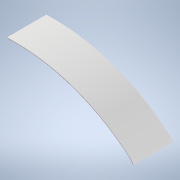
# Autodesk Inventor part: Hood Lexan
Saved by Autodesk Inventor 2022 (Build 260153070, 153G)
## iProperties
Created: 2021-09-03
Part Number: Hood Lexan
Material: Polycarbonate, Clear
Document SubType Name: Modeling
Designer: Main Account
Density: 1.2 g/cm^3
Appearance: Polycarbonate - Clear
Author: Main Account
Autodesk Inventor part; units mm, degrees
ref_plane "YZ Plane" through (0, 0, 0) normal (1, 0, 0) x (0, 1, 0)
ref_plane "XZ Plane" through (0, 0, 0) normal (0, 1, 0) x (-1, 0, 0)
ref_plane "XY Plane" through (0, 0, 0) normal (0, 0, 1) x (1, 0, 0)
sketch "Sketch1" plane through (0, 0, 0) normal (0, 0, 1) x (1, 0, 0)
  line L0 (6.4002, -1.3978) -> (19.527, -1.3978)
  line L1 (6.4002, -1.3978) -> (6.4002, -2.9853)
  line L2 (6.4002, -2.9853) -> (19.527, -2.9853)
  line L3 (333.1851, -123.7146) -> (327.4784, -114.9672)
  line L4 (333.1851, -123.7146) -> (331.8555, -124.582)
  line L5 (331.8555, -124.582) -> (326.1488, -115.8346)
  arc A0 (327.4784, -114.9672) -> (19.527, -1.3978) centre (26.9726, -455.509) ccw
  arc A1 (326.1488, -115.8346) -> (19.527, -2.9853) centre (26.4701, -457.1045) ccw
  point P0 (0, 0)
  dimension "d1" = 1.5875
  dimension "d2" = 1.5875
  dimension "d3" = 454.1723
  constraints: 12 end point, 4 point on circle, 2 centre point, 2 horizontal, 1 perpendicular, 1 vertical
  measures "d1" distance of L0.start L1.end
  measures "d2" distance of L3.end L5.end
  measures "d3" radius of A1
extrude "Extrusion1" add sketch "Sketch1" against normal blind 101.6
body "Solid1"
